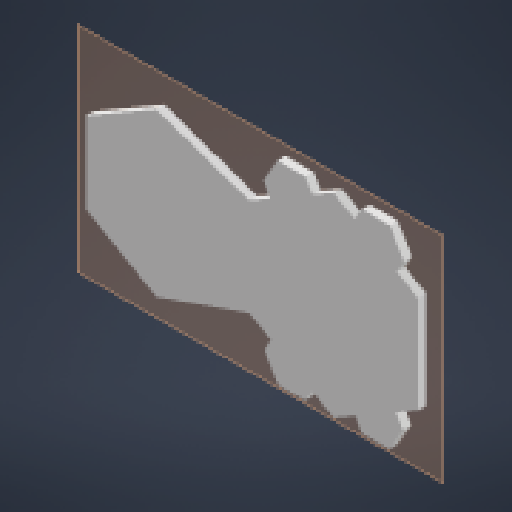
# Autodesk Inventor part: Base_STABLE
Saved by Autodesk Inventor 2025.3 (Build 293356000, 356)
## iProperties
Created: 2025-04-18
Part Number: Base_STABLE
Material: Generic
Document SubType Name: Modeling
Designer: Nelson
Density: 1 g/cm^3
Appearance: Default
Author: Nelson
Autodesk Inventor part; units mm, degrees
ref_plane "YZ Plane" through (0, 0, 0) normal (1, 0, 0) x (0, 1, 0)
ref_plane "XZ Plane" through (0, 0, 0) normal (0, 1, 0) x (-1, 0, 0)
sketch "Sketch1" plane through (0, 0, 0) normal (0, 0, 1) x (1, 0, 0)
  line L0 (0, 50) -> (43.3013, 25)
  line L1 (43.3013, 25) -> (43.3013, -25)
  line L2 (43.3013, -25) -> (0, -50)
  line L3 (0, -50) -> (-43.3013, -25)
  line L4 (-43.3013, -25) -> (-43.3013, 25)
  line L5 (-43.3013, 25) -> (0, 50)
  line L6 (0, 0) -> (109.27, 0)
  line L7 (109.27, 60) -> (161.2315, 30)
  line L8 (161.2315, 30) -> (161.2315, -30)
  line L9 (161.2315, -30) -> (109.27, -60)
  line L10 (109.27, -60) -> (57.3085, -30)
  line L11 (57.3085, -30) -> (57.3085, 30)
  line L12 (57.3085, 30) -> (109.27, 60)
  line L13 (143.911, 60) -> (152.5713, 45)
  line L14 (152.5713, 45) -> (143.911, 30)
  line L15 (143.911, 30) -> (126.5905, 30)
  line L16 (126.5905, 30) -> (117.9303, 45)
  line L17 (117.9303, 45) -> (126.5905, 60)
  line L18 (126.5905, 60) -> (143.911, 60)
  line L19 (74.629, 60) -> (91.9495, 60)
  line L20 (91.9495, 60) -> (100.6097, 45)
  line L21 (100.6097, 45) -> (91.9495, 30)
  line L22 (91.9495, 30) -> (74.629, 30)
  line L23 (74.629, 30) -> (65.9687, 45)
  line L24 (65.9687, 45) -> (74.629, 60)
  line L25 (74.9307, -59.4774) -> (66.5722, -45)
  line L26 (66.5722, -45) -> (74.9307, -30.5226)
  line L27 (74.9307, -30.5226) -> (91.6478, -30.5226)
  line L28 (91.6478, -30.5226) -> (100.0063, -45)
  line L29 (100.0063, -45) -> (91.6478, -59.4774)
  line L30 (91.6478, -59.4774) -> (74.9307, -59.4774)
  line L31 (143.6093, -59.4774) -> (126.8922, -59.4774)
  line L32 (126.8922, -59.4774) -> (118.5337, -45)
  line L33 (118.5337, -45) -> (126.8922, -30.5226)
  line L34 (126.8922, -30.5226) -> (143.6093, -30.5226)
  line L35 (143.6093, -30.5226) -> (151.9678, -45)
  line L36 (151.9678, -45) -> (143.6093, -59.4774)
  line L37 (57.3085, 30) -> (0, 50)
  line L38 (0, -50) -> (57.3085, -30)
  circle A0 centre (109.27, 0) radius 10
  point P0 (135.2508, 45)
  point P1 (83.2892, 45)
  point P2 (83.2892, -45)
  point P3 (135.2508, -45)
  point P4 (70.7514, -37.7613)
  point P5 (95.827, -52.2387)
  point P6 (122.713, -52.2387)
  point P7 (147.7886, -37.7613)
  point P8 (148.2411, 37.5)
  point P9 (122.2604, 52.5)
  point P10 (96.2796, 52.5)
  point P11 (70.2989, 37.5)
  dimension "d0" = 50
  dimension "d1" = 109.27
  dimension "d2" = 60
  dimension "d5" = 20
  constraints: 78 end point, 4 midpoint, 3 coincident, 1 centre point, 1 horizontal, 1 point on line, 78 other
  measures "d0" distance of L0.start point (0, 0)
  measures "d1" distance of L6.start L6.end
  measures "d2" distance of L6.end L7.start
  measures "d5" diameter of A0
extrude "Extrusion1" add sketch "Sketch1" along normal blind 5 contours L37 L11 L6 L1 L0 | L0 L1 L2 L3 L4 L5 | L12 L23 L22 L21 L20 L7 L17 L16 L15 L14 L8 L9 L35 L34 L33 L32 L10 L29 L28 L27 L26 L11 | L6 L11 L38 L2 L1 | L23 L24 L19 L20 L12 | L12 L20 L21 L22 L23 | L26 L27 L28 L29 L10 | L10 L29 L30 L25 L26 | L17 L18 L13 L14 L7 | L7 L14 L15 L16 L17 | L32 L33 L34 L35 L9 | L9 L35 L36 L31 L32 | A0
extrude "Extrusion2" cut sketch "Sketch1" along normal blind 5 contours A0
equation "\"d6\" = L_Plate"
equation "\"L_Plate\" = 5"
body "Solid1"
